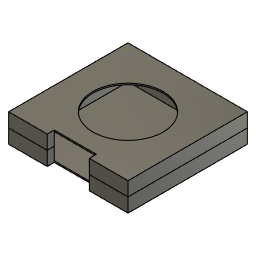
camera case v2 (Autodesk Fusion 360 design; units mm, degrees)
Autodesk Fusion 360 part; units mm, degrees
sketch "Sketch1" plane through (0, 0, 0) normal (0, 1, 0) x (1, 0, 0)
  line L0 (-50, 50) -> (35, 50)
  line L1 (35, 50) -> (35, -35)
  line L2 (35, -35) -> (-50, -35)
  line L3 (-50, -35) -> (-50, 50)
  line L4 (30, -30) -> (-45, -30)
  line L5 (-45, -30) -> (-45, 45)
  line L6 (-45, 45) -> (30, 45)
  line L7 (30, 45) -> (30, -30)
  line L8 (-7.5, -30) -> (2.5, -30)
  line L9 (-7.5, -30) -> (-17.5, -30)
  line L10 (2.5, -30) -> (2.5, -35)
  line L11 (-17.5, -30) -> (-17.5, -35)
  circle A0 centre (-7.5, 7.5) radius 25
  dimension "d1" = 5
  dimension "d6" = 10
  dimension "d7" = 10
  dimension "d13" = 50
  constraint horizontal L0
  constraint vertical L1
  constraint horizontal L2
  constraint vertical L3
  constraint midpoint L4 L8.start
  constraint parallel L4 L8
  constraint parallel L4 L9
  constraint coincident L2 L10.end
  constraint perpendicular L2 L10
  constraint perpendicular L4 L11
  measures "d6" distance of L8.start L8.end
  measures "d7" distance of L8.start L9.end
  measures "d13" diameter of A0
extrude "Extrude1" add sketch "Sketch1" along normal blind 10 contours L0 L1 L2 L3 L4 L5 L6 L7 L10 L11 | L2 L4 L8 L9 L10 L11 makes body 1
extrude "Extrude2" add sketch "Sketch1" along normal blind 1 contours L4 L5 L6 L7 L8 L9 | A0 bodies 1
extrude "Extrude3" cut sketch "Sketch1" along normal blind 10 contours L2 L4 L8 L9 L10 L11 bodies 1
ref_plane "WorkPlane1" through (-7.5, 10, -7.5) normal (0, 1, 0) x (0, 0, 1)
mirror "Mirror1" about plane through (-7.5, 10, -7.5) normal (0, 1, 0) of bodies 1 merged
extrude "Extrude4" cut sketch "Sketch1" along normal blind 10 contours A0 bodies 1
extrude "Extrude5" cut 1 faces at (2.5, 7, 33.3333) along direction (1, 0, 0) blind 5 on bodies 1 bodies 1
extrude "Extrude6" cut 1 faces at (-17.5, 7, 33.3333) along direction (-1, 0, 0) blind 5 on bodies 1 bodies 1
split "Split1" by plane through (-7.5, 10, -7.5) normal (0, 1, 0) bodies 1 makes body 2 at (-12.5, 20, -23.3333)
move_body "Move1" bodies 2 1 to x (-1, 0, 0) y (0, -1, 0) z (0, 0, 1) at (3.7836, 40, 0)
